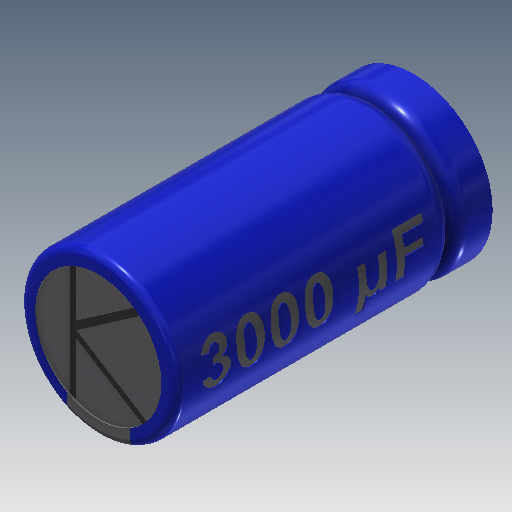
# Autodesk Inventor part: config - capasitor 3000 μF
Saved by Autodesk Inventor 2019.1 (Build 231200000, 200)
## iProperties
Company: Autodesk Asia Pte. Ltd.
Created: 2005-12-06
Part Number: config - capasitor 3000 μF
Document SubType Name: Modeling
Designer: Simon.Ng@autodesk.com
Stock Number: config - capasitor 3000 μF
Density: 1 g/cm^3
Material: Generic
Mass: 1.55363 g
Surface Area: 7.94542 cm^2
Volume: 1.55363 cm^3
Appearance: Blue - Wall Paint - Glossy
Title: PC Demo
Author: Simon.Ng@autodesk.com
Autodesk Inventor part; units mm, degrees
ref_plane "YZ Plane" through (0, 0, 0) normal (1, 0, 0) x (0, 1, 0)
ref_plane "XZ Plane" through (0, 0, 0) normal (0, 1, 0) x (-1, 0, 0)
ref_plane "XY Plane" through (0, 0, 0) normal (0, 0, 1) x (1, 0, 0)
sketch "Sketch1" plane through (0, 0, 0) normal (0, 0, 1) x (1, 0, 0)
  line L0 (0, 8) -> (0, -6) construction
  line L1 (-6, 0) -> (8, 0) construction
  circle A0 centre (0, 0) radius 5
  dimension "d0" = 10
  constraints: 2 point on line, 1 centre point
  measures "d0" diameter of A0
extrude "Extrusion1" add sketch "Sketch1" along normal blind 20
sketch "Sketch6" plane through (0, 0, 0) normal (1, 0, 0) x (0, 1, 0)
  line L0 (0, 29.25) -> (0, -2.25) projected
  line L1 (5, 0) -> (5, 20) projected
  line L2 (5, 3.5) -> (5, 1.5)
  line L3 (5, 2.5) -> (4.5, 2.5) construction
  line L4 (-5, 0) -> (5, 0) construction
  arc A0 (4.5, 2.5) -> (5, 3.5) centre (3.75, 3.5) ccw
  arc A1 (5, 1.5) -> (4.5, 2.5) centre (3.75, 1.5) ccw
  point P0 (0, 0)
  dimension "d16" = 2
  dimension "d17" = 2.5
  dimension "d18" = 0.5
  constraints: 4 end point, 4 point on circle, 2 centre point, 2 point on line, 2 tangent, 1 collinear, 1 horizontal, 1 midpoint
  measures "d16" distance of L2.start L2.end
  measures "d17" distance between parallel lines of L4 L3
  measures "d18" distance of L3.start L3.end
revolve "Revolution1" cut sketch "Sketch6" angle 360 about axis through (0, 0, 0) along (0, 0, -1)
sketch "Sketch2" plane through (0, 0, 20) normal (0, 0, 1) x (1, 0, 0)
  circle A0 centre (0, 0) radius 5 projected
  circle A1 centre (0, 0) radius 4
  dimension "d3" = 1
  constraints: 1 centre point, 1 coincident
  measures "d3" radial gap between concentric circles of A1 A0
extrude "Extrusion2" cut sketch "Sketch2" against normal blind 0.1 contours A1
sketch "Sketch3" plane through (0, 0, 19.9) normal (0, 0, 1) x (1, 0, 0)
  line L0 (-1.9077, 3.7158) -> (-1.4809, 3.7158)
  line L1 (-1.4809, 3.7158) -> (-1.4809, -3.8634)
  line L2 (-1.4809, -3.8634) -> (-1.9077, -3.8634)
  line L3 (-1.9077, -3.8634) -> (-1.9077, 3.7158)
  line L4 (-1.4809, 0.1279) -> (-1.7316, 0.4886)
  line L5 (-1.7316, 0.4886) -> (2.5228, 3.4459)
  line L6 (2.5228, 3.4459) -> (2.7735, 3.0852)
  line L7 (2.7735, 3.0852) -> (-1.4809, 0.1279)
  line L8 (-1.4809, 0.1279) -> (-1.6828, -0.1969)
  line L9 (-1.6828, -0.1969) -> (2.9946, -3.106)
  line L10 (2.9946, -3.106) -> (3.1965, -2.7813)
  line L11 (3.1965, -2.7813) -> (-1.4809, 0.1279)
  circle A0 centre (0, 0) radius 4 projected
  constraints: 24 end point, 6 parallel, 3 perpendicular, 1 horizontal, 1 point on line, 2 other
extrude "Extrusion3" cut sketch "Sketch3" against normal blind 0.05 contours L0 A0 L3 | L1 L5 L4 L8 L9 A0 L3 | L5 A0 L7 L1 | L1 L4 L5 | L5 L6 L7 A0 | A0 L1 L2 L3 | L11 A0 L9 L1 | L1 L9 L8 | L11 L10 L9 A0
fillet "Fillet1" radius 0.5 1 edges at (-5, 0, 20)
sketch "Sketch5" plane through (0, 0, 20) normal (0, 0, 1) x (1, 0, 0)
  circle A0 centre (0, 0) radius 4 projected
  circle A1 centre (0, 0) radius 5 projected
  line L0 (2, -3.4641) -> (2, -6)
  line L1 (2, -6) -> (-2, -6)
  line L2 (-2, -6) -> (-2, -3.4641)
  line L3 (0, -6) -> (0, 8) projected
  point P0 (0, -5)
  point P1 (0, -5)
  dimension "d12" = 1
  dimension "d13" = 4
  constraints: 6 end point, 2 point on circle, 1 coincident, 1 parallel, 1 point on line, 1 vertical alignment, 2 other
  measures "d12" distance from line of L1 point (0, -5)
  measures "d13" distance of L0.end L1.end
split_face "Split1"
ref_plane "Work Plane1" through (10, 0, 0) normal (1, 0, 0) x (0, 1, 0)
sketch "Sketch4" plane through (10, 0, 0) normal (1, 0, 0) x (0, 0, -1)
  line L0 (-18.5356, 1.8542) -> (-2.9274, 1.8542) construction
  line L1 (-2.9274, 1.8542) -> (-2.9274, -1.985) construction
  line L2 (-2.9274, -1.985) -> (-18.5356, -1.985) construction
  line L3 (-18.5356, -1.985) -> (-18.5356, 1.8542) construction
  line L4 (-18.3883, -0.2117) -> (-17.8697, -0.1476)
  spline S0 degree 3 poles (-17.8697, -0.1476) (-17.8441, -0.3461) (-17.6264, -0.5574) (-17.4728, -0.5574) knots 0 0 0 0 1 1 1 1
  spline S1 degree 3 poles (-17.4728, -0.5574) (-17.3063, -0.5574) (-17.0801, -0.3056) (-17.0801, -0.0922) knots 0 0 0 0 1 1 1 1
  spline S2 degree 3 poles (-17.0801, -0.0922) (-17.0801, 0.1106) (-17.2957, 0.3475) (-17.4514, 0.3475) knots 0 0 0 0 1 1 1 1
  spline S3 degree 2 poles (-17.4514, 0.3475) (-17.5539, 0.3475) (-17.6969, 0.3069) knots 0 0 0 1 1 1
  line L5 (-17.6969, 0.3069) -> (-17.6371, 0.7444)
  spline S4 degree 3 poles (-17.6371, 0.7444) (-17.4194, 0.738) (-17.1911, 0.9386) (-17.1911, 1.1051) knots 0 0 0 0 1 1 1 1
  spline S5 degree 3 poles (-17.1911, 1.1051) (-17.1911, 1.246) (-17.3597, 1.4124) (-17.4984, 1.4124) knots 0 0 0 0 1 1 1 1
  spline S6 degree 3 poles (-17.4984, 1.4124) (-17.6371, 1.4124) (-17.8313, 1.2225) (-17.8527, 1.0389) knots 0 0 0 0 1 1 1 1
  line L6 (-17.8527, 1.0389) -> (-18.3478, 1.1222)
  spline S7 degree 4 poles (-18.3478, 1.1222) (-18.2966, 1.3761) (-18.0874, 1.6813) (-17.7161, 1.8542) (-17.4835, 1.8542) knots 0 0 0 0 0 1 1 1 1 1
  spline S8 degree 2 poles (-17.4835, 1.8542) (-17.0886, 1.8542) (-16.8496, 1.6024) knots 0 0 0 1 1 1
  spline S9 degree 2 poles (-16.8496, 1.6024) (-16.6533, 1.3975) (-16.6533, 1.1371) knots 0 0 0 1 1 1
  spline S10 degree 2 poles (-16.6533, 1.1371) (-16.6533, 0.77) (-17.0566, 0.5502) knots 0 0 0 1 1 1
  spline S11 degree 3 poles (-17.0566, 0.5502) (-16.8155, 0.499) (-16.5295, 0.1383) (-16.5295, -0.1156) knots 0 0 0 0 1 1 1 1
  spline S12 degree 3 poles (-16.5295, -0.1156) (-16.5295, -0.4848) (-17.0673, -1.0034) (-17.4685, -1.0034) knots 0 0 0 0 1 1 1 1
  spline S13 degree 3 poles (-17.4685, -1.0034) (-17.8484, -1.0034) (-18.3478, -0.5659) (-18.3883, -0.2117) knots 0 0 0 0 1 1 1 1
  spline S14 degree 2 poles (-15.2874, 1.8542) (-14.8798, 1.8542) (-14.6514, 1.5639) knots 0 0 0 1 1 1
  spline S15 degree 2 poles (-14.6514, 1.5639) (-14.3783, 1.2203) (-14.3783, 0.4243) knots 0 0 0 1 1 1
  spline S16 degree 2 poles (-14.3783, 0.4243) (-14.3783, -0.3696) (-14.6536, -0.7175) knots 0 0 0 1 1 1
  spline S17 degree 2 poles (-14.6536, -0.7175) (-14.8798, -1.0034) (-15.2874, -1.0034) knots 0 0 0 1 1 1
  spline S18 degree 3 poles (-15.2874, -1.0034) (-15.6972, -1.0034) (-16.1966, -0.376) (-16.1966, 0.4307) knots 0 0 0 0 1 1 1 1
  spline S19 degree 2 poles (-16.1966, 0.4307) (-16.1966, 1.2203) (-15.9213, 1.5682) knots 0 0 0 1 1 1
  spline S20 degree 2 poles (-15.9213, 1.5682) (-15.695, 1.8542) (-15.2874, 1.8542) knots 0 0 0 1 1 1
  spline S21 degree 3 poles (-15.2874, 1.4082) (-15.3856, 1.4082) (-15.5371, 1.2844) (-15.5798, 1.1243) knots 0 0 0 0 1 1 1 1
  spline S22 degree 2 poles (-15.5798, 1.1243) (-15.6353, 0.9173) (-15.6353, 0.4243) knots 0 0 0 1 1 1
  spline S23 degree 4 poles (-15.6353, 0.4243) (-15.6353, -0.0665) (-15.535, -0.4357) (-15.3856, -0.5574) (-15.2874, -0.5574) knots 0 0 0 0 0 1 1 1 1 1
  spline S24 degree 3 poles (-15.2874, -0.5574) (-15.1893, -0.5574) (-15.0377, -0.4336) (-14.995, -0.2736) knots 0 0 0 0 1 1 1 1
  spline S25 degree 2 poles (-14.995, -0.2736) (-14.9396, -0.0665) (-14.9396, 0.4243) knots 0 0 0 1 1 1
  spline S26 degree 4 poles (-14.9396, 0.4243) (-14.9396, 0.9173) (-15.0399, 1.2844) (-15.1893, 1.4082) (-15.2874, 1.4082) knots 0 0 0 0 0 1 1 1 1 1
  spline S27 degree 2 poles (-13.1127, 1.8542) (-12.7051, 1.8542) (-12.4768, 1.5639) knots 0 0 0 1 1 1
  spline S28 degree 2 poles (-12.4768, 1.5639) (-12.2036, 1.2203) (-12.2036, 0.4243) knots 0 0 0 1 1 1
  spline S29 degree 2 poles (-12.2036, 0.4243) (-12.2036, -0.3696) (-12.4789, -0.7175) knots 0 0 0 1 1 1
  spline S30 degree 2 poles (-12.4789, -0.7175) (-12.7051, -1.0034) (-13.1127, -1.0034) knots 0 0 0 1 1 1
  spline S31 degree 3 poles (-13.1127, -1.0034) (-13.5225, -1.0034) (-14.0219, -0.376) (-14.0219, 0.4307) knots 0 0 0 0 1 1 1 1
  spline S32 degree 2 poles (-14.0219, 0.4307) (-14.0219, 1.2203) (-13.7466, 1.5682) knots 0 0 0 1 1 1
  spline S33 degree 2 poles (-13.7466, 1.5682) (-13.5204, 1.8542) (-13.1127, 1.8542) knots 0 0 0 1 1 1
  spline S34 degree 3 poles (-13.1127, 1.4082) (-13.2109, 1.4082) (-13.3624, 1.2844) (-13.4051, 1.1243) knots 0 0 0 0 1 1 1 1
  spline S35 degree 2 poles (-13.4051, 1.1243) (-13.4606, 0.9173) (-13.4606, 0.4243) knots 0 0 0 1 1 1
  spline S36 degree 4 poles (-13.4606, 0.4243) (-13.4606, -0.0665) (-13.3603, -0.4357) (-13.2109, -0.5574) (-13.1127, -0.5574) knots 0 0 0 0 0 1 1 1 1 1
  spline S37 degree 3 poles (-13.1127, -0.5574) (-13.0146, -0.5574) (-12.863, -0.4336) (-12.8204, -0.2736) knots 0 0 0 0 1 1 1 1
  spline S38 degree 2 poles (-12.8204, -0.2736) (-12.7649, -0.0665) (-12.7649, 0.4243) knots 0 0 0 1 1 1
  spline S39 degree 4 poles (-12.7649, 0.4243) (-12.7649, 0.9173) (-12.8652, 1.2844) (-13.0146, 1.4082) (-13.1127, 1.4082) knots 0 0 0 0 0 1 1 1 1 1
  spline S40 degree 2 poles (-10.938, 1.8542) (-10.5304, 1.8542) (-10.3021, 1.5639) knots 0 0 0 1 1 1
  spline S41 degree 2 poles (-10.3021, 1.5639) (-10.0289, 1.2203) (-10.0289, 0.4243) knots 0 0 0 1 1 1
  spline S42 degree 2 poles (-10.0289, 0.4243) (-10.0289, -0.3696) (-10.3042, -0.7175) knots 0 0 0 1 1 1
  spline S43 degree 2 poles (-10.3042, -0.7175) (-10.5304, -1.0034) (-10.938, -1.0034) knots 0 0 0 1 1 1
  spline S44 degree 3 poles (-10.938, -1.0034) (-11.3478, -1.0034) (-11.8472, -0.376) (-11.8472, 0.4307) knots 0 0 0 0 1 1 1 1
  spline S45 degree 2 poles (-11.8472, 0.4307) (-11.8472, 1.2203) (-11.5719, 1.5682) knots 0 0 0 1 1 1
  spline S46 degree 2 poles (-11.5719, 1.5682) (-11.3457, 1.8542) (-10.938, 1.8542) knots 0 0 0 1 1 1
  spline S47 degree 3 poles (-10.938, 1.4082) (-11.0362, 1.4082) (-11.1877, 1.2844) (-11.2304, 1.1243) knots 0 0 0 0 1 1 1 1
  spline S48 degree 2 poles (-11.2304, 1.1243) (-11.2859, 0.9173) (-11.2859, 0.4243) knots 0 0 0 1 1 1
  spline S49 degree 4 poles (-11.2859, 0.4243) (-11.2859, -0.0665) (-11.1856, -0.4357) (-11.0362, -0.5574) (-10.938, -0.5574) knots 0 0 0 0 0 1 1 1 1 1
  spline S50 degree 3 poles (-10.938, -0.5574) (-10.8399, -0.5574) (-10.6883, -0.4336) (-10.6457, -0.2736) knots 0 0 0 0 1 1 1 1
  spline S51 degree 2 poles (-10.6457, -0.2736) (-10.5902, -0.0665) (-10.5902, 0.4243) knots 0 0 0 1 1 1
  spline S52 degree 4 poles (-10.5902, 0.4243) (-10.5902, 0.9173) (-10.6905, 1.2844) (-10.8399, 1.4082) (-10.938, 1.4082) knots 0 0 0 0 0 1 1 1 1 1
  line L7 (-8.4752, 1.0731) -> (-7.9374, 1.0731)
  line L8 (-7.9374, 1.0731) -> (-7.9374, 0.1511)
  spline S53 degree 4 poles (-7.9374, 0.1511) (-7.9374, -0.1071) (-7.8841, -0.3973) (-7.6963, -0.5766) (-7.5639, -0.5766) knots 0 0 0 0 0 1 1 1 1 1
  spline S54 degree 4 poles (-7.5639, -0.5766) (-7.4274, -0.5766) (-7.2289, -0.3888) (-7.1713, -0.122) (-7.1713, 0.1447) knots 0 0 0 0 0 1 1 1 1 1
  line L9 (-7.1713, 0.1447) -> (-7.1713, 1.0731)
  line L10 (-7.1713, 1.0731) -> (-6.6335, 1.0731)
  line L11 (-6.6335, 1.0731) -> (-6.6335, -0.9565)
  line L12 (-6.6335, -0.9565) -> (-7.1286, -0.9565)
  line L13 (-7.1286, -0.9565) -> (-7.1286, -0.7111)
  spline S55 degree 2 poles (-7.1286, -0.7111) (-7.278, -1.0013) (-7.5362, -1.0013) knots 0 0 0 1 1 1
  spline S56 degree 2 poles (-7.5362, -1.0013) (-7.8094, -1.0013) (-7.9374, -0.7111) knots 0 0 0 1 1 1
  line L14 (-7.9374, -0.7111) -> (-7.9374, -1.729)
  line L15 (-7.9374, -1.729) -> (-8.4752, -1.729)
  line L16 (-8.4752, -1.729) -> (-8.4752, 1.0731)
  line L17 (-6.0722, -0.9565) -> (-6.0722, 1.8435)
  line L18 (-6.0722, 1.8435) -> (-4.1493, 1.8435)
  line L19 (-4.1493, 1.8435) -> (-4.1493, 1.3697)
  line L20 (-4.1493, 1.3697) -> (-5.5066, 1.3697)
  line L21 (-5.5066, 1.3697) -> (-5.5066, 0.7082)
  line L22 (-5.5066, 0.7082) -> (-4.335, 0.7082)
  line L23 (-4.335, 0.7082) -> (-4.335, 0.2344)
  line L24 (-4.335, 0.2344) -> (-5.5066, 0.2344)
  line L25 (-5.5066, 0.2344) -> (-5.5066, -0.9565)
  line L26 (-5.5066, -0.9565) -> (-6.0722, -0.9565)
  constraints: 2 other
emboss "Emboss1" sketch "Sketch4" operation cut depth 0.05 direction (1, 0, 0) wrap yes faces at (-0.6132, 4.9623, 8.8333) (-0.6132, 4.9623, 8.8333) (-0.6132, 4.9623, 8.8333) (-0.6132, 4.9623, 1) (-0.6132, 4.9623, 1) (-0.6132, 4.9623, 1) (-0.6132, 4.9623, 1) (-0.6132, 4.9623, 8.8333)
body "Solid1"
